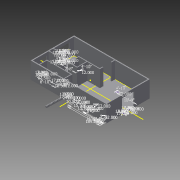
# Autodesk Inventor part: West_Test_Structure_2nd_Floor_Devices
Saved by Autodesk Inventor 2013 SP2 (Build 170200200, 200)
## iProperties
Created: 2013-07-10
Part Number: West_Test_Structure_2nd_Floor_Devices
Material: Generic
Document SubType Name: Modeling
Designer: jmw3
Density: 1 g/cm^3
Author: jmw3
Autodesk Inventor part; units mm, degrees
ref_plane "YZ Plane" through (0, 0, 0) normal (1, 0, 0) x (0, 1, 0)
ref_plane "XZ Plane" through (0, 0, 0) normal (0, 1, 0) x (-1, 0, 0)
ref_plane "XY Plane" through (0, 0, 0) normal (0, 0, 1) x (1, 0, 0)
sketch "Sketch1" plane through (0, 0, 0) normal (0, 0, 1) x (1, 0, 0)
  line L0 (-5588, 3200.4) -> (5588, 3200.4)
  line L1 (5588, -3200.4) -> (-5588, -3200.4)
  line L2 (-3958.3754, 3048) -> (-719.8754, 3048)
  line L3 (5435.6, 914.4) -> (5588, 914.4)
  line L4 (5588, -914.4) -> (5435.6, -914.4)
  line L5 (-4072.6754, 3048) -> (-605.5754, 3048)
  line L6 (5588, 3200.4) -> (5588, 914.4)
  line L7 (5588, -914.4) -> (5588, -3200.4)
  line L8 (5435.6, 3048) -> (5435.6, 914.4)
  line L9 (5435.6, -914.4) -> (5435.6, -3048)
  line L10 (-5588, 894.5564) -> (-5588, 3200.4)
  line L11 (-5435.6, 76.2) -> (-5435.6, 3048)
  line L12 (0, -4480.56) -> (0, 4480.56) projected
  line L13 (-7823.2, 0) -> (7823.2, 0) projected
  line L14 (-863.6, -3048) -> (-863.6, -2006.6)
  line L15 (-863.6, -2006.6) -> (-4381.5, -2006.6)
  line L16 (-4495.8, -2006.6) -> (-4495.8, -3048)
  line L17 (-5435.6, 76.2) -> (-3581.4, 76.2)
  line L18 (-3581.4, 76.2) -> (-3581.4, -685.8)
  line L19 (-3581.4, -685.8) -> (-5435.6, -685.8)
  line L20 (-5435.6, -571.5) -> (-5435.6, -38.1)
  line L21 (-5435.6, -38.1) -> (-3695.7, -38.1)
  line L22 (-3695.7, -38.1) -> (-3695.7, -571.5)
  line L23 (-3695.7, -571.5) -> (-5435.6, -571.5)
  line L24 (-5435.6, -571.5) -> (-5435.6, -38.1)
  line L25 (-5588, -965.2) -> (-5435.6, -965.2)
  line L26 (-5435.6, -1879.6) -> (-5588, -1879.6)
  line L27 (-5435.6, -3048) -> (-5435.6, -1879.6)
  line L28 (-5588, -3200.4) -> (-5588, -1879.6)
  line L29 (-5588, -965.2) -> (-5588, 914.4)
  line L30 (-2590.8, 914.4) -> (-1377.4097, 914.4)
  line L31 (-1244.6, 800.1) -> (-1244.6, -685.8)
  line L32 (-1244.6, -685.8) -> (-2590.8, -685.8)
  line L33 (-2590.8, -685.8) -> (-2590.8, 914.4)
  line L34 (-1377.4097, 914.4) -> (508, 914.4)
  line L35 (622.3, 952.5) -> (622.3, 800.1)
  line L36 (622.3, 800.1) -> (-1244.6, 800.1)
  line L37 (508, 914.4) -> (508, 1314.45)
  line L38 (508, 1314.45) -> (622.3, 1314.45)
  line L39 (622.3, 1314.45) -> (622.3, 800.1)
  line L40 (622.3, 3048) -> (622.3, 2533.65)
  line L41 (622.3, 2533.65) -> (508, 2533.65)
  line L42 (508, 2533.65) -> (508, 3048)
  line L43 (-2476.5, 800.1) -> (-1358.9, 800.1)
  line L44 (-1358.9, 800.1) -> (-1358.9, -571.5)
  line L45 (-1358.9, -571.5) -> (-2476.5, -571.5)
  line L46 (-2476.5, -571.5) -> (-2476.5, 800.1)
  line L47 (-749.3, -3048) -> (-749.3, -1892.3)
  line L48 (-749.3, -1892.3) -> (-4495.8, -1892.3)
  line L49 (-4495.8, -1892.3) -> (-4495.8, -2006.6)
  line L50 (-5435.6, 3048) -> (508, 3048)
  line L51 (622.3, 3048) -> (5435.6, 3048)
  line L52 (-4381.5, -2006.6) -> (-4381.5, -3048)
  line L53 (-863.6, -2006.6) -> (-1060.3581, -2006.6)
  line L54 (-5435.6, -965.2) -> (-5435.6, -685.8)
  line L55 (-5435.6, -571.5) -> (-5435.6, -38.1)
  line L56 (-4495.8, -3048) -> (-5435.6, -3048)
  line L57 (5435.6, -3048) -> (-749.3, -3048)
  line L58 (-863.6, -3048) -> (-4381.5, -3048)
  line L59 (880.3246, -3048) -> (-749.3, -3048)
  line L60 (-5435.6, -38.1) -> (-5435.6, -571.5)
  line L61 (-5435.6, -685.8) -> (-5435.6, -965.2)
  line L62 (-5435.6, -685.8) -> (-3581.4, -685.8)
  line L63 (-5435.6, 76.2) -> (-3581.4, 76.2)
  line L64 (-5435.6, 76.2) -> (-5435.6, 3048)
  line L65 (-5435.6, -685.8) -> (-5435.6, -965.2)
  line L66 (-5435.6, -965.2) -> (-5588, -965.2)
  line L67 (-5588, -965.2) -> (-5588, 3200.4)
  line L68 (-5435.6, 3048) -> (-5435.6, 76.2)
  line L69 (-5435.6, 76.2) -> (-3581.4, 76.2)
  line L70 (-3581.4, 76.2) -> (-3581.4, -685.8)
  line L71 (-3581.4, -685.8) -> (-5435.6, -685.8)
  line L72 (-5435.6, -571.5) -> (-3695.7, -571.5)
  line L73 (-3695.7, -571.5) -> (-3695.7, -38.1)
  line L74 (-3695.7, -38.1) -> (-5435.6, -38.1)
  line L75 (-5435.6, -38.1) -> (-5435.6, -571.5)
  dimension "d14" = 1828.8
  dimension "d90" = 6299.2
  dimension "d94" = 114.3
  dimension "d95" = 114.3
  dimension "d96" = 114.3
  dimension "d99" = 914.4
  dimension "d100" = 152.4
  dimension "d102" = 939.8
  dimension "d104" = 990.6
  dimension "d105" = 114.3
  dimension "d106" = 114.3
  dimension "d107" = 114.3
  dimension "d108" = 114.3
  dimension "d109" = 114.3
  dimension "d110" = 6680.2
  dimension "d112" = 1219.2
  dimension "d120" = 152.4
  dimension "d122" = 2971.8
  dimension "d123" = 2286
  dimension "d124" = 5943.6
  dimension "d125" = 114.3
  dimension "d127" = 114.3
  dimension "d128" = 6400.8
  dimension "d129" = 152.4
  dimension "d130" = 1168.4
  dimension "d131" = 1041.4
  dimension "d132" = 114.3
  dimension "d133" = 1854.2
  dimension "d134" = 2362.2
  dimension "d135" = 10871.2
  dimension "d236" = 2133.6
  dimension "d237" = 514.35
  dimension "d238" = 114.3
  constraints: 148 end point, 38 parallel, 28 perpendicular, 26 collinear, 12 horizontal, 3 point on line, 3 other
  measures "d14" distance between parallel lines of L4 L3
  measures "d90" distance between parallel lines of L9 L14
  measures "d94" distance between parallel lines of L19 L23
  measures "d95" distance between parallel lines of L18 L22
  measures "d96" distance between parallel lines of L17 L21
  measures "d99" distance between parallel lines of L25 L26
  measures "d100" distance between parallel lines of L10 L11
  measures "d102" distance between parallel lines of L27 L16
  measures "d104" distance between parallel lines of L18 L33
  measures "d105" distance between parallel lines of L33 L46
  measures "d106" distance between parallel lines of L31 L44
  measures "d107" distance between parallel lines of L32 L45
  measures "d108" distance between parallel lines of L30 L43
  measures "d109" distance between parallel lines of L39 L37
  measures "d110" distance between parallel lines of L8 L31
  measures "d112" distance from line of L38.end L41
  measures "d120" distance between parallel lines of L50 L0
  measures "d122" distance between parallel lines of L50 L17
  measures "d123" distance between parallel lines of L1 L4
  measures "d124" distance between parallel lines of L11 L37
  measures "d125" distance between parallel lines of L16 L52
  measures "d127" distance between parallel lines of L14 L47
  measures "d128" distance between parallel lines of L1 L0
  measures "d129" distance between parallel lines of L1 L57
  measures "d130" distance between parallel lines of L56 L26
  measures "d131" distance between parallel lines of L58 L15
  measures "d132" distance between parallel lines of L15 L48
  measures "d133" distance between parallel lines of L54 L18
  measures "d134" distance between parallel lines of L56 L19
  measures "d135" distance between parallel lines of L9 L27
  measures "d236" distance between parallel lines of L50 L30
  measures "d237" distance between parallel lines of L36 L38
  measures "d238" distance of L40.end L41.end
extrude "Extrusion7" add sketch "Sketch1" along normal blind 2463.8 contours L57 L9 L4 L7 L1 L12 | L12 L1 L28 L26 L27 L56 L16 L49 L48 L47 L57 | L0 L12 L50 L5 L2 L11 L17 L18 L13 L29 L10 | L0 L6 L3 L8 L51 L40 L41 L42 L50 L12 | L34 L37 L38 L39 L35 L36 L12 | L12 L36 L31 L13 L44 L43 L46 L33 L30 L34 | L13 L18 L19 L54 L25 L29 | L13 L46 L45 L44 L31 L32 L33
sketch "Sketch4" plane through (0, 0, 0) normal (0, 0, -1) x (-1, 0, 0)
  line L0 (4381.5, -3048) -> (863.6, -3048) projected
  line L1 (863.6, -3048) -> (863.6, -2006.6) projected
  line L2 (863.6, -2006.6) -> (4381.5, -2006.6) projected
  line L3 (4381.5, -2006.6) -> (4381.5, -3048) projected
  line L4 (-5435.6, -3048) -> (749.3, -3048) projected
  line L5 (-5435.6, -914.4) -> (-5435.6, -3048) projected
  line L6 (-5588, -914.4) -> (-5435.6, -914.4) projected
  line L7 (-5588, -3200.4) -> (-5588, -914.4) projected
  line L8 (5588, -3200.4) -> (-5588, -3200.4) projected
  line L9 (5588, -1879.6) -> (5588, -3200.4) projected
  line L10 (5435.6, -1879.6) -> (5588, -1879.6) projected
  line L11 (5435.6, -3048) -> (5435.6, -1879.6) projected
  line L12 (4495.8, -3048) -> (5435.6, -3048) projected
  line L13 (4495.8, -1892.3) -> (4495.8, -3048) projected
  line L14 (749.3, -1892.3) -> (4495.8, -1892.3) projected
  line L15 (749.3, -3048) -> (749.3, -1892.3) projected
  line L16 (3695.7, -571.5) -> (3695.7, -38.1) projected
  line L17 (3695.7, -38.1) -> (5435.6, -38.1) projected
  line L18 (5435.6, -38.1) -> (5435.6, -571.5) projected
  line L19 (5435.6, -571.5) -> (3695.7, -571.5) projected
  line L20 (5435.6, 3048) -> (-508, 3048) projected
  line L21 (5435.6, 76.2) -> (5435.6, 3048) projected
  line L22 (3581.4, 76.2) -> (5435.6, 76.2) projected
  line L23 (3581.4, -685.8) -> (3581.4, 76.2) projected
  line L24 (5435.6, -685.8) -> (3581.4, -685.8) projected
  line L25 (5435.6, -965.2) -> (5435.6, -685.8) projected
  line L26 (5588, -965.2) -> (5435.6, -965.2) projected
  line L27 (5588, 3200.4) -> (5588, -965.2) projected
  line L28 (-5588, 3200.4) -> (5588, 3200.4) projected
  line L29 (-5588, 914.4) -> (-5588, 3200.4) projected
  line L30 (-5435.6, 914.4) -> (-5588, 914.4) projected
  line L31 (-5435.6, 3048) -> (-5435.6, 914.4) projected
  line L32 (-622.3, 3048) -> (-5435.6, 3048) projected
  line L33 (-622.3, 2533.65) -> (-622.3, 3048) projected
  line L34 (-508, 2533.65) -> (-622.3, 2533.65) projected
  line L35 (-508, 3048) -> (-508, 2533.65) projected
  line L36 (1358.9, -571.5) -> (1358.9, 800.1) projected
  line L37 (1358.9, 800.1) -> (2476.5, 800.1) projected
  line L38 (2476.5, 800.1) -> (2476.5, -571.5) projected
  line L39 (2476.5, -571.5) -> (1358.9, -571.5) projected
  line L40 (2590.8, 914.4) -> (-508, 914.4) projected
  line L41 (-508, 914.4) -> (-508, 1314.45) projected
  line L42 (-508, 1314.45) -> (-622.3, 1314.45) projected
  line L43 (-622.3, 1314.45) -> (-622.3, 800.1) projected
  line L44 (-622.3, 800.1) -> (1244.6, 800.1) projected
  line L45 (1244.6, 800.1) -> (1244.6, -685.8) projected
  line L46 (1244.6, -685.8) -> (2590.8, -685.8) projected
  line L47 (2590.8, -685.8) -> (2590.8, 914.4) projected
  line L48 (-5588, 3200.4) -> (5588, 3200.4)
  line L49 (5588, 3200.4) -> (5588, -2006.6)
  line L50 (5588, -2006.6) -> (-5588, -2006.6)
  line L51 (-5588, -2006.6) -> (-5588, 3200.4)
  line L52 (-5588, -2006.6) -> (863.6, -2006.6)
  line L53 (863.6, -2006.6) -> (863.6, -3200.4)
  line L54 (863.6, -3200.4) -> (-5588, -3200.4)
  line L55 (-5588, -3200.4) -> (-5588, -2006.6)
  line L56 (4381.5, -2006.6) -> (5588, -2006.6)
  line L57 (5588, -2006.6) -> (5588, -3200.4)
  line L58 (5588, -3200.4) -> (4381.5, -3200.4)
  line L59 (4381.5, -3200.4) -> (4381.5, -2006.6)
  line L60 (4381.5, -3048) -> (863.6, -3048)
  line L61 (863.6, -3048) -> (863.6, -3200.4)
  line L62 (863.6, -3200.4) -> (4381.5, -3200.4)
  line L63 (4381.5, -3200.4) -> (4381.5, -3048)
  line L64 (863.6, -3200.4) -> (4381.5, -3200.4)
  line L65 (4381.5, -3200.4) -> (4381.5, -2895.6)
  line L66 (4381.5, -2895.6) -> (863.6, -2895.6)
  line L67 (863.6, -2895.6) -> (863.6, -3200.4)
  point P0 (0, 0)
  dimension "d192" = 889
  constraints: 40 end point, 10 parallel, 5 horizontal, 5 perpendicular, 3 point on line
  measures "d192" distance between parallel lines of L66 L2
extrude "Extrusion8" add sketch "Sketch4" against normal blind 25.4 contours L59 L8 L53 L0 | L3 L50 L13 L12 L11 L9 L8 L59 | L53 L8 L7 L50 L5 L4 L15 L1 | L2 L50 L15 L14 L13 | L50 L11 L12 L13 | L13 L14 L15 L50 L5 L6 L51 L30 L31 L32 L33 L34 L35 L20 L21 L22 L23 L24 L25 L26 L49 L10 L11 | L50 L11 L10 L9 | L15 L4 L5 L50 | L7 L6 L5 L50 | L26 L25 L24 L23 L22 L21 L20 L35 L34 L33 L32 L31 L30 L29 L28 L27 | L16 L17 L18 L19 | L36 L37 L38 L39 | L47 L46 L45 L44 L43 L42 L41 L40
sketch "Sketch5" plane through (-749.3, -3048, 2463.8) normal (1, 0, 0) x (0, 0, -1)
  line L0 (2438.4, 0) -> (2438.4, 1155.7) projected
  line L1 (2438.4, 1155.7) -> (0, 1155.7) projected
  line L2 (2438.4, 114.3) -> (406.4, 114.3)
  line L3 (406.4, 114.3) -> (406.4, 927.1)
  line L4 (406.4, 927.1) -> (2438.4, 927.1)
  line L5 (2438.4, 927.1) -> (2438.4, 114.3)
  line L6 (2438.4, 165.1) -> (457.2, 165.1)
  line L7 (457.2, 165.1) -> (457.2, 876.3)
  line L8 (457.2, 876.3) -> (2438.4, 876.3)
  line L9 (2438.4, 876.3) -> (2438.4, 165.1)
  point P0 (2463.8, 3048)
  dimension "d140" = 2032
  dimension "d142" = 228.6
  dimension "d143" = 812.8
  dimension "d144" = 1981.2
  dimension "d145" = 711.2
  dimension "d146" = 50.8
  constraints: 16 end point, 4 parallel, 2 horizontal, 2 perpendicular, 2 point on line
  measures "d140" distance between parallel lines of L5 L3
  measures "d142" distance between parallel lines of L1 L4
  measures "d143" distance between parallel lines of L4 L2
  measures "d144" distance between parallel lines of L9 L7
  measures "d145" distance between parallel lines of L6 L8
  measures "d146" distance between parallel lines of L2 L6
extrude "Extrusion9" cut sketch "Sketch5" against normal blind 50.8 contours L2 L3 L4 L0 L8 L7 L6
extrude "Extrusion10" cut sketch "Sketch5" against normal up to surface (114.3 mm away) contours L6 L7 L8 L0
sketch "Sketch6" plane through (0, 0, 2463.8) normal (0, 0, 1) x (1, 0, 0)
  line L0 (-3695.7, -38.1) -> (-3695.7, -571.5) projected
  line L1 (-3695.7, -571.5) -> (-5435.6, -571.5) projected
  line L2 (-5435.6, -571.5) -> (-5435.6, -38.1) projected
  line L3 (-5435.6, -38.1) -> (-3695.7, -38.1) projected
  line L4 (-5435.6, 3048) -> (508, 3048) projected
  line L5 (508, 3048) -> (508, 2533.65) projected
  line L6 (508, 2533.65) -> (622.3, 2533.65) projected
  line L7 (622.3, 2533.65) -> (622.3, 3048) projected
  line L8 (622.3, 3048) -> (5435.6, 3048) projected
  line L9 (5435.6, 3048) -> (5435.6, 914.4) projected
  line L10 (5435.6, 914.4) -> (5588, 914.4) projected
  line L11 (5588, 914.4) -> (5588, 3200.4) projected
  line L12 (5588, 3200.4) -> (-5588, 3200.4) projected
  line L13 (-5588, 3200.4) -> (-5588, -965.2) projected
  line L14 (-5588, -965.2) -> (-5435.6, -965.2) projected
  line L15 (-5435.6, -965.2) -> (-5435.6, -685.8) projected
  line L16 (-5435.6, -685.8) -> (-3581.4, -685.8) projected
  line L17 (-3581.4, -685.8) -> (-3581.4, 76.2) projected
  line L18 (-3581.4, 76.2) -> (-5435.6, 76.2) projected
  line L19 (-5435.6, 76.2) -> (-5435.6, 3048) projected
  line L20 (-1358.9, 800.1) -> (-1358.9, -571.5) projected
  line L21 (-1358.9, -571.5) -> (-2476.5, -571.5) projected
  line L22 (-2476.5, -571.5) -> (-2476.5, 800.1) projected
  line L23 (-2476.5, 800.1) -> (-1358.9, 800.1) projected
  line L24 (508, 914.4) -> (-2590.8, 914.4) projected
  line L25 (-2590.8, 914.4) -> (-2590.8, -685.8) projected
  line L26 (-2590.8, -685.8) -> (-1244.6, -685.8) projected
  line L27 (-1244.6, -685.8) -> (-1244.6, 800.1) projected
  line L28 (-1244.6, 800.1) -> (622.3, 800.1) projected
  line L29 (622.3, 800.1) -> (622.3, 1314.45) projected
  line L30 (622.3, 1314.45) -> (508, 1314.45) projected
  line L31 (508, 1314.45) -> (508, 914.4) projected
  line L32 (5435.6, 914.4) -> (5588, 914.4)
  line L33 (5588, 914.4) -> (5588, -914.4)
  line L34 (5588, -914.4) -> (5435.6, -914.4)
  line L35 (5435.6, -914.4) -> (5435.6, 914.4)
  line L36 (-5588, -965.2) -> (-5435.6, -965.2)
  line L37 (-5435.6, -965.2) -> (-5435.6, -1879.6)
  line L38 (-5435.6, -1879.6) -> (-5588, -1879.6)
  line L39 (-5588, -1879.6) -> (-5588, -965.2)
  point P0 (0, 0)
  constraints: 16 end point, 4 parallel, 2 horizontal, 2 perpendicular
extrude "Extrusion11" add sketch "Sketch6" against normal blind 406.4 contours L37 L38 L39 L14 | L10 L33 L34 L35
sketch "Sketch7" plane through (-5435.6, 76.2, 2463.8) normal (1, 0, 0) x (0, 0, -1)
  line L0 (2438.4, 0) -> (2438.4, 2971.8) projected
  line L1 (2438.4, 2971.8) -> (0, 2971.8) projected
  line L2 (431.8, 647.7) -> (1346.2, 647.7)
  line L3 (1346.2, 647.7) -> (1346.2, 2324.1)
  line L4 (1346.2, 2324.1) -> (431.8, 2324.1)
  line L5 (431.8, 2324.1) -> (431.8, 647.7)
  point P0 (2463.8, -76.2)
  dimension "d153" = 1676.4
  dimension "d155" = 914.4
  dimension "d156" = 1092.2
  dimension "d157" = 647.7
  constraints: 8 end point, 2 parallel, 1 horizontal, 1 perpendicular
  measures "d153" distance between parallel lines of L2 L4
  measures "d155" distance between parallel lines of L5 L3
  measures "d156" distance between parallel lines of L0 L3
  measures "d157" distance between parallel lines of L1 L4
extrude "Extrusion12" cut sketch "Sketch7" against normal up to surface (152.4 mm away)
sketch "Sketch9" plane through (-863.6, -3048, 2463.8) normal (-1, 0, 0) x (0, 0, 1)
  line L0 (-2463.8, 0) -> (-2438.4, 0)
  line L1 (-2438.4, 0) -> (-2438.4, 152.4)
  line L2 (-2438.4, 152.4) -> (-2463.8, 152.4)
  line L3 (-2463.8, 152.4) -> (-2463.8, 0)
  point P0 (-2463.8, 3048)
  dimension "d193" = 152.4
  constraints: 8 end point, 2 parallel, 1 horizontal, 1 perpendicular
  measures "d193" distance between parallel lines of L2 L0
extrude "Extrusion14" add sketch "Sketch9" along normal up to surface (3517.9 mm away)
sketch "Sketch11" plane through (0, 0, 2057.4) normal (0, 0, -1) x (-1, 0, 0)
  line L0 (-5435.6, -914.4) -> (-5435.6, 914.4) projected
  line L1 (-5588, 914.4) -> (-5588, -914.4) projected
  line L2 (7823.2, 0) -> (-7823.2, 0) projected
  line L3 (-5588, 12.7) -> (-5435.6, 12.7)
  line L4 (-5435.6, 12.7) -> (-5435.6, -12.7)
  line L5 (-5435.6, -12.7) -> (-5588, -12.7)
  line L6 (-5588, -12.7) -> (-5588, 12.7)
  point P0 (0, 0)
  dimension "d230" = 25.4
  constraints: 8 end point, 2 parallel, 2 point on line, 1 horizontal, 1 perpendicular, 1 other
  measures "d230" distance between parallel lines of L5 L3
extrude "Extrusion16" add sketch "Sketch11" along normal blind 25.4
sketch "Sketch10" plane through (-4381.5, -2006.6, 2463.8) normal (0, -1, 0) x (1, 0, 0)
  line L0 (3517.9, -2463.8) -> (3517.9, 0) projected
  line L1 (0, 0) -> (3517.9, 0) projected
  line L2 (3632.2, -2438.4) -> (-114.3, -2438.4) projected
  line L3 (-114.3, -2438.4) -> (-114.3, 0) projected
  line L4 (3632.2, 0) -> (-114.3, 0) projected
  line L5 (3632.2, -2438.4) -> (3632.2, 0) projected
  line L6 (850.9, -5016.5) -> (1041.4, -5016.5)
  line L7 (1041.4, -5016.5) -> (1041.4, -4832.35)
  line L8 (1041.4, -4832.35) -> (914.4, -4832.35)
  line L9 (1041.4, -4832.35) -> (1231.9, -4832.35)
  line L10 (1231.9, -4832.35) -> (1231.9, -4648.2)
  line L11 (1231.9, -4648.2) -> (1041.4, -4648.2)
  line L12 (1041.4, -4648.2) -> (1041.4, -4832.35)
  line L13 (1612.9, -4464.05) -> (1612.9, -4279.9)
  line L14 (1422.4, -4648.2) -> (1422.4, -4464.05)
  line L15 (1422.4, -4464.05) -> (1612.9, -4464.05)
  line L16 (1612.9, -4279.9) -> (1422.4, -4279.9)
  line L17 (1422.4, -4279.9) -> (1422.4, -4464.05)
  line L18 (1231.9, -4648.2) -> (1422.4, -4648.2)
  line L19 (1422.4, -4464.05) -> (1231.9, -4464.05)
  line L20 (1231.9, -4464.05) -> (1231.9, -4648.2)
  line L21 (2184.4, -3911.6) -> (2184.4, -3727.45)
  line L22 (2184.4, -3543.3) -> (2184.4, -3727.45)
  line L23 (2184.4, -3727.45) -> (2374.9, -3727.45)
  line L24 (2374.9, -3543.3) -> (2184.4, -3543.3)
  line L25 (1993.9, -3727.45) -> (1993.9, -3911.6)
  line L26 (1993.9, -3911.6) -> (2184.4, -3911.6)
  line L27 (2184.4, -3727.45) -> (1993.9, -3727.45)
  line L28 (2374.9, -3727.45) -> (2374.9, -3543.3)
  line L29 (1993.9, -4095.75) -> (1993.9, -3911.6)
  line L30 (1993.9, -3911.6) -> (1803.4, -3911.6)
  line L31 (1803.4, -4095.75) -> (1993.9, -4095.75)
  line L32 (1803.4, -3911.6) -> (1803.4, -4095.75)
  line L33 (1803.4, -4279.9) -> (1803.4, -4095.75)
  line L34 (1803.4, -4095.75) -> (1612.9, -4095.75)
  line L35 (1612.9, -4279.9) -> (1803.4, -4279.9)
  line L36 (1612.9, -4095.75) -> (1612.9, -4279.9)
  line L37 (2755.9, -3175) -> (2946.4, -3175)
  line L38 (2946.4, -3175) -> (2946.4, -2990.85)
  line L39 (2946.4, -2806.7) -> (2946.4, -2990.85)
  line L40 (2946.4, -2990.85) -> (3136.9, -2990.85)
  line L41 (3136.9, -2806.7) -> (2946.4, -2806.7)
  line L42 (3136.9, -2990.85) -> (3136.9, -2806.7)
  line L43 (3136.9, -2622.55) -> (3136.9, -2806.7)
  line L44 (3136.9, -2806.7) -> (3327.4, -2806.7)
  line L45 (3327.4, -2622.55) -> (3136.9, -2622.55)
  line L46 (3327.4, -2806.7) -> (3327.4, -2622.55)
  line L47 (2374.9, -3359.15) -> (2374.9, -3543.3)
  line L48 (2374.9, -3543.3) -> (2565.4, -3543.3)
  line L49 (2565.4, -3543.3) -> (2565.4, -3359.15)
  line L50 (2565.4, -3359.15) -> (2374.9, -3359.15)
  line L51 (2565.4, -3175) -> (2565.4, -3359.15)
  line L52 (2565.4, -3359.15) -> (2755.9, -3359.15)
  line L53 (2755.9, -3175) -> (2565.4, -3175)
  line L54 (2755.9, -3359.15) -> (2755.9, -3175)
  line L55 (2755.9, -2990.85) -> (2755.9, -3175)
  line L56 (2946.4, -2990.85) -> (2755.9, -2990.85)
  line L57 (3327.4, -2622.55) -> (3517.9, -2622.55)
  line L58 (3517.9, -2622.55) -> (3517.9, -2438.4)
  line L59 (3517.9, -2438.4) -> (3327.4, -2438.4)
  line L60 (3327.4, -2438.4) -> (3327.4, -2622.55)
  line L61 (3136.9, -2762.25) -> (3327.4, -2762.25)
  line L62 (1041.4, -4832.35) -> (850.9, -4832.35)
  line L63 (850.9, -4832.35) -> (850.9, -5016.5)
  line L64 (1041.4, -5016.5) -> (1041.4, -4832.35)
  line L65 (850.9, -5016.5) -> (660.4, -5016.5)
  line L66 (660.4, -5016.5) -> (660.4, -5200.65)
  line L67 (660.4, -5200.65) -> (850.9, -5200.65)
  line L68 (850.9, -5200.65) -> (850.9, -5016.5)
  point P0 (4381.5, -2463.8)
  dimension "d197" = 184.15
  dimension "d198" = 190.5
  dimension "d199" = 184.15
  dimension "d200" = 190.5
  dimension "d201" = 184.15
  dimension "d202" = 190.5
  dimension "d203" = 184.15
  dimension "d204" = 190.5
  dimension "d205" = 184.15
  dimension "d206" = 190.5
  dimension "d207" = 184.15
  dimension "d208" = 190.5
  dimension "d209" = 184.15
  dimension "d210" = 190.5
  dimension "d211" = 184.15
  dimension "d212" = 190.5
  dimension "d213" = 184.15
  dimension "d214" = 190.5
  dimension "d215" = 184.15
  dimension "d216" = 190.5
  dimension "d217" = 184.15
  dimension "d218" = 190.5
  dimension "d219" = 184.15
  dimension "d220" = 190.5
  dimension "d221" = 184.15
  dimension "d222" = 184.15
  dimension "d223" = 190.5
  dimension "d224" = 190.5
  dimension "d225" = 190.5
  dimension "d226" = 184.15
  constraints: 127 end point, 31 parallel, 16 horizontal, 16 perpendicular, 14 collinear, 2 point on line
  measures "d197" distance between parallel lines of L8 L6
  measures "d198" distance between parallel lines of L10 L12
  measures "d199" distance between parallel lines of L11 L9
  measures "d200" distance between parallel lines of L20 L14
  measures "d201" distance between parallel lines of L19 L18
  measures "d202" distance between parallel lines of L13 L17
  measures "d203" distance between parallel lines of L16 L15
  measures "d204" distance between parallel lines of L36 L33
  measures "d205" distance between parallel lines of L34 L35
  measures "d206" distance between parallel lines of L29 L32
  measures "d207" distance between parallel lines of L30 L31
  measures "d208" distance between parallel lines of L25 L21
  measures "d209" distance between parallel lines of L27 L26
  measures "d210" distance between parallel lines of L28 L22
  measures "d211" distance between parallel lines of L24 L23
  measures "d212" distance between parallel lines of L49 L47
  measures "d213" distance between parallel lines of L50 L48
  measures "d214" distance between parallel lines of L51 L54
  measures "d215" distance between parallel lines of L53 L52
  measures "d216" distance between parallel lines of L38 L55
  measures "d217" distance between parallel lines of L56 L37
  measures "d218" distance between parallel lines of L39 L42
  measures "d219" distance between parallel lines of L41 L40
  measures "d220" distance between parallel lines of L46 L43
  measures "d221" distance between parallel lines of L45 L44
  measures "d222" distance between parallel lines of L57 L59
  measures "d223" distance between parallel lines of L60 L58
  measures "d224" distance between parallel lines of L63 L64
  measures "d225" distance between parallel lines of L68 L66
  measures "d226" distance between parallel lines of L65 L67
extrude "Extrusion15" add sketch "Sketch10" along normal blind 889 contours L58 L57 L60 L2 L0 | L68 L67 L66 L65 | L7 L6 L63 L62 L8 | L10 L9 L12 L11 | L14 L18 L20 L19 | L13 L15 L17 L16 | L33 L35 L36 L34 | L29 L31 L32 L30 | L21 L26 L25 L27 | L28 L23 L22 L24 | L49 L48 L47 L50 | L54 L52 L51 L53 | L38 L37 L55 L56 | L42 L40 L39 L41 | L46 L61 L43 L45
sketch "Sketch12" plane through (0, 0, 25.4) normal (0, 0, 1) x (1, 0, 0)
  line L0 (-1054.1, -2895.6) -> (-863.6, -2895.6)
  line L1 (-863.6, -2895.6) -> (-863.6, -2006.6)
  line L2 (-863.6, -2006.6) -> (-1054.1, -2006.6)
  line L3 (-1054.1, -2006.6) -> (-1054.1, -2895.6)
  point P0 (0, 0)
  constraints: 8 end point, 2 parallel, 1 horizontal, 1 perpendicular
extrude "Extrusion17" cut sketch "Sketch12" against normal blind 0.0254
sketch "Sketch13" plane through (0, 0, 25.4) normal (0, 0, 1) x (1, 0, 0)
  line L0 (-863.6, -2171.7) -> (-863.6, -2882.9) projected
  line L1 (5435.6, -3048) -> (-749.3, -3048) projected
  line L2 (5435.6, -914.4) -> (5435.6, -3048) projected
  line L3 (5588, -914.4) -> (5435.6, -914.4) projected
  line L4 (5435.6, 914.4) -> (5588, 914.4) projected
  line L5 (5435.6, 3048) -> (5435.6, 914.4) projected
  line L6 (622.3, 3048) -> (5435.6, 3048) projected
  line L7 (-5435.6, 3048) -> (508, 3048) projected
  line L8 (-5435.6, 76.2) -> (-5435.6, 3048) projected
  line L9 (-3581.4, -685.8) -> (-3581.4, 76.2) projected
  line L10 (-5435.6, -965.2) -> (-5435.6, -685.8) projected
  line L11 (-5588, -965.2) -> (-5435.6, -965.2) projected
  line L12 (-5588, -965.2) -> (-5588, -1879.6) projected
  line L13 (-5435.6, -1879.6) -> (-5588, -1879.6) projected
  line L14 (-5435.6, -3048) -> (-5435.6, -1879.6) projected
  line L15 (-749.3, -1892.3) -> (-4495.8, -1892.3) projected
  line L16 (-749.3, -2120.9) -> (-749.3, -1892.3) projected
  circle A0 centre (-5435.6, -1422.4) radius 152.4
  line L17 (-5219.7, -1638.3) -> (-5651.5, -1638.3)
  circle A1 centre (-863.6, -2527.3) radius 152.4
  line L18 (-647.7, -2743.2) -> (-1079.5, -2743.2)
  line L19 (-1079.5, -2743.2) -> (-1079.5, -2311.4)
  circle A2 centre (406.4, -2527.3) radius 152.4
  circle A3 centre (4368.8, -2438.4) radius 152.4
  circle A4 centre (-3098.8, 1574.8) radius 152.4
  circle A5 centre (2387.6, -1524) radius 152.4
  circle A6 centre (2387.6, 1574.8) radius 152.4
  circle A7 centre (-5588, 1841.5) radius 152.4
  line L20 (-5372.1, 1625.6) -> (-5803.9, 1625.6)
  line L21 (-5803.9, 1625.6) -> (-5803.9, 2057.4)
  line L22 (-5803.9, 2057.4) -> (-5372.1, 1625.6)
  line L23 (-5586.4125, -963.6125) -> (-5586.4125, -965.2)
  circle A8 centre (5435.6, 457.2) radius 152.4
  line L24 (5651.5, 241.3) -> (5219.7, 241.3)
  line L25 (5219.7, 673.1) -> (5651.5, 241.3)
  line L26 (5219.7, 241.3) -> (5219.7, 673.1)
  line L27 (-7899.4, 0) -> (7835.9, 0) projected
  line L28 (0, -4480.56) -> (0, 4480.56) projected
  line L29 (-1079.5, -2311.4) -> (-647.7, -2743.2)
  line L30 (-5651.5, -1638.3) -> (-5651.5, -1206.5)
  line L31 (-5651.5, -1206.5) -> (-5219.7, -1638.3)
  line L32 (-5588, 723.9) -> (-5588, 2400.3) projected
  line L33 (-5435.6, 723.9) -> (-5588, 723.9) projected
  line L34 (-5435.6, 2400.3) -> (-5435.6, 723.9) projected
  line L35 (-5435.6, 2400.3) -> (-5588, 2400.3) projected
  circle A9 centre (-5588, 1282.7) radius 152.4
  line L36 (-5372.1, 1066.8) -> (-5803.9, 1066.8)
  line L37 (-5803.9, 1498.6) -> (-5372.1, 1066.8)
  line L38 (-5803.9, 1066.8) -> (-5803.9, 1498.6)
  circle A10 centre (-2743.2, -1422.4) radius 152.4
  line L39 (-3314.7, -1206.5) -> (-2882.9, -1206.5)
  line L40 (-2882.9, -1206.5) -> (-2882.9, -1638.3)
  line L41 (-2882.9, -1638.3) -> (-3314.7, -1638.3)
  line L42 (-3314.7, -1638.3) -> (-3314.7, -1206.5)
  line L43 (190.5, -2222.5) -> (622.3, -2222.5)
  line L44 (622.3, -2222.5) -> (622.3, -2654.3)
  line L45 (622.3, -2654.3) -> (190.5, -2654.3)
  line L46 (190.5, -2654.3) -> (190.5, -2222.5)
  circle A11 centre (2387.6, -2438.4) radius 152.4
  line L47 (2603.5, -2654.3) -> (2171.7, -2654.3)
  line L48 (2171.7, -2654.3) -> (2171.7, -2222.5)
  line L49 (2171.7, -2222.5) -> (2603.5, -2654.3)
  line L50 (5219.7, -673.1) -> (5219.7, -241.3)
  line L51 (5219.7, -241.3) -> (5651.5, -673.1)
  line L52 (5651.5, -673.1) -> (5219.7, -673.1)
  circle A12 centre (5435.6, -457.2) radius 152.4
  line L53 (2563.5764, -2133.6) -> (2739.5527, -2438.4)
  line L54 (2739.5527, -2438.4) -> (2563.5764, -2743.2)
  line L55 (2563.5764, -2743.2) -> (2211.6236, -2743.2)
  line L56 (2211.6236, -2743.2) -> (2035.6473, -2438.4)
  line L57 (2035.6473, -2438.4) -> (2211.6236, -2133.6)
  line L58 (2211.6236, -2133.6) -> (2563.5764, -2133.6)
  line L59 (-687.6236, -2222.5) -> (-511.6473, -2527.3)
  line L60 (-511.6473, -2527.3) -> (-687.6236, -2832.1)
  line L61 (-687.6236, -2832.1) -> (-1039.5764, -2832.1)
  line L62 (-1039.5764, -2832.1) -> (-1215.5527, -2527.3)
  line L63 (-1215.5527, -2527.3) -> (-1039.5764, -2222.5)
  line L64 (-1039.5764, -2222.5) -> (-687.6236, -2222.5)
  point P0 (0, 0)
  point P1 (5435.6, -457.2)
  point P2 (5435.6, 457.2)
  point P3 (-863.6, -2222.5)
  dimension "d242" = 304.8
  dimension "d246" = 457.2
  dimension "d247" = 431.8
  dimension "d248" = 431.8
  dimension "d249" = 241.3
  dimension "d251" = 304.8
  dimension "d252" = 431.8
  dimension "d253" = 431.8
  dimension "d256" = 215.9
  dimension "d257" = 304.8
  dimension "d258" = 304.8
  dimension "d259" = 304.8
  dimension "d260" = 304.8
  dimension "d261" = 304.8
  dimension "d262" = 304.8
  dimension "d263" = 431.8
  dimension "d264" = 431.8
  dimension "d265" = 215.9
  dimension "d266" = 304.8
  dimension "d267" = 431.8
  dimension "d268" = 431.8
  dimension "d269" = 215.9
  dimension "d270" = 1473.2
  dimension "d271" = 2336.8
  dimension "d272" = 1473.2
  dimension "d273" = 3048
  dimension "d274" = 1524
  dimension "d275" = 3048
  dimension "d276" = 5029.2
  dimension "d277" = 1066.8
  dimension "d278" = 609.6
  dimension "d280" = 215.9
  dimension "d281" = 558.8
  dimension "d282" = 304.8
  dimension "d283" = 431.8
  dimension "d284" = 431.8
  dimension "d285" = 215.9
  dimension "d286" = 558.8
  dimension "d287" = 304.8
  dimension "d289" = 2692.4
  dimension "d290" = 431.8
  dimension "d291" = 431.8
  dimension "d292" = 215.9
  dimension "d293" = 2120.9
  dimension "d294" = 431.8
  dimension "d295" = 431.8
  dimension "d296" = 393.7
  dimension "d297" = 4813.3
  dimension "d298" = 304.8
  dimension "d299" = 609.6
  dimension "d300" = 3048
  dimension "d301" = 431.8
  dimension "d302" = 431.8
  dimension "d303" = 393.7
  dimension "d304" = 304.8
  dimension "d305" = 431.8
  dimension "d306" = 431.8
  dimension "d307" = 215.9
  dimension "d308" = 457.2
  dimension "d309" = 457.2
  dimension "d310" = 609.6
  dimension "d311" = 609.6
  dimension "d332" = 469.9
  dimension "d333" = 520.7
  constraints: 84 end point, 19 parallel, 13 centre point, 10 midpoint, 7 point on line, 2 coincident, 2 horizontal, 2 perpendicular, 26 other
  measures "d242" diameter of A0
  measures "d246" distance from line of L13 A0.centre
  measures "d247" distance of L17.end L30.end
  measures "d248" distance of L17.start L17.end
  measures "d249" distance between parallel lines of L13 L17
  measures "d251" diameter of A1
  measures "d252" distance of L18.start L18.end
  measures "d253" distance of L18.end L19.end
  measures "d256" distance between parallel lines of L0 L19
  measures "d257" diameter of A2
  measures "d258" diameter of A3
  measures "d259" diameter of A4
  measures "d260" diameter of A5
  measures "d261" diameter of A6
  measures "d262" diameter of A7
  measures "d263" distance of L20.end L22.start
  measures "d264" distance of L20.start L20.end
  measures "d265" distance from line of A7.centre L21
  measures "d266" diameter of A8
  measures "d267" distance of L26.start L26.end
  measures "d268" distance of L25.end L26.start
  measures "d269" distance from line of A8.centre L26
  measures "d270" distance from line of L7 A4.centre
  measures "d271" distance from line of L8 A4.centre
  measures "d272" distance from line of L6 A6.centre
  measures "d273" distance from line of L5 A6.centre
  measures "d274" distance from line of L1 A5.centre
  measures "d275" distance from line of L2 A5.centre
  measures "d276" distance from line of L2 A2.centre
  measures "d277" distance from line of L2 A3.centre
  measures "d278" distance from line of L1 A3.centre
  measures "d280" distance from line of A0.centre L30
  measures "d281" distance from line of L35 A7.centre
  measures "d282" diameter of A9
  measures "d283" distance of L36.end L38.end
  measures "d284" distance of L36.start L36.end
  measures "d285" distance from line of A9.centre L38
  measures "d286" distance from line of L33 A9.centre
  measures "d287" diameter of A10
  measures "d289" distance from line of L14 A10.centre
  measures "d290" distance of L41.end L39.start
  measures "d291" distance of L39.start L39.end
  measures "d292" distance from line of A10.centre L39
  measures "d293" distance between parallel lines of L14 L42
  measures "d294" distance between parallel lines of L43 L45
  measures "d295" distance of L43.start L43.end
  measures "d296" distance between parallel lines of L1 L45
  measures "d297" distance between parallel lines of L2 L44
  measures "d298" diameter of A11
  measures "d299" distance from line of L1 A11.centre
  measures "d300" distance from line of L2 A11.centre
  measures "d301" distance of L47.end L48.end
  measures "d302" distance of L47.start L47.end
  measures "d303" distance between parallel lines of L1 L47
  measures "d304" diameter of A12
  measures "d305" distance of L50.start L50.end
  measures "d306" distance of L51.end L50.start
  measures "d307" distance from line of A12.centre L50
  measures "d308" distance from line of L3 A12.centre
  measures "d309" distance from line of L4 A8.centre
  measures "d310" distance between parallel lines of L55 L58
  measures "d311" distance between parallel lines of L61 L64
  measures "d332" distance from line of L15 A10.centre
  measures "d333" distance from line of L1 A2.centre
extrude "Extrusion18" add sketch "Sketch13" along normal blind 76.2 contours A1 L29 L0 | L0 L29 A1 | L29 A1 L0 | L0 A1 L29 | A7 L22 L32 | L32 L22 A7 | A7 L32 L22 | L22 L32 A7 | A9 L37 L32 | L32 L37 A9 | A9 L32 L37 | L32 A9 L37 | A0 L31 | A0 L31 | A2 L45 | L45 A2 | A3 | A4 | A5 | A6 | A8 L25 | L25 A8 | A10 L40 | L40 A10 | A11 L49 | L49 A11 | A12 L51 | L51 A12
extrude "Extrusion19" add sketch "Sketch13" along normal blind 50.8 contours L29 A1 L0 | L0 A1 L29 | A1 L0 L18 L19 L29 | A1 L29 L18 L0 | L22 L20 L8 | L8 L20 L32 A7 L22 | A7 L32 L22 | L22 L32 A7 | A7 L32 L20 L21 L22 | L37 L36 L8 | L8 L36 L32 A9 L37 | A9 L32 L37 | L32 A9 L37 | A9 L32 L36 L38 L37 | L31 A0 L12 | L12 L17 L30 L31 | A0 L31 L17 L12 | A0 L31 | A2 L45 | A2 L45 L46 L43 L44 | L25 A8 | A8 L25 L24 L26 | L40 A10 | A10 L40 L41 L42 L39 | L49 A11 | A11 L49 L47 L48 | L50 L51 A12 L52 | L51 A12 picked at (-796.0057, -2602.9381) picked at (-952.3828, -2576.3685) picked at (-5529.2995, 1758.7694) picked at (-5626.8195, 1747.7815) picked at (-5529.2995, 1199.9694) picked at (-5626.8195, 1188.9815) picked at (-5481.3692, -1400.3587) picked at (366.3236, -2477.213) picked at (5377.7074, 448.3062) picked at (-2884.7373, -1406.9827) picked at (2347.883, -2478.5688) picked at (5377.7074, -466.0938)
extrude "Extrusion20" add sketch "Sketch13" along normal blind 25.4 contours L64 L59 L60 L61 L0 L18 L29 A1 | L0 A1 L29 L19 L18 L61 L62 L63 L64 | L53 L54 L55 L56 L57 L58
sketch "Sketch15" plane through (-5435.6, 723.9, 1117.6) normal (0, 0, 1) x (1, 0, 0)
  line L0 (-152.4, 0) -> (-152.4, 1676.4) projected
  line L1 (0, 0) -> (-152.4, 0) projected
  line L2 (0, 1676.4) -> (-152.4, 1676.4) projected
  circle A0 centre (-152.4, 1117.6) radius 152.4
  line L3 (63.5, 901.7) -> (-368.3, 901.7)
  line L4 (-368.3, 1333.5) -> (63.5, 901.7)
  line L5 (-368.3, 901.7) -> (-368.3, 1333.5)
  line L6 (63.5, 342.9) -> (-368.3, 342.9)
  circle A1 centre (-152.4, 558.8) radius 152.4
  line L7 (-368.3, 342.9) -> (-368.3, 774.7)
  line L8 (-368.3, 774.7) -> (63.5, 342.9)
  point P0 (5435.6, -723.9)
  dimension "d318" = 304.8
  dimension "d319" = 431.8
  dimension "d320" = 431.8
  dimension "d321" = 215.9
  dimension "d322" = 304.8
  dimension "d323" = 431.8
  dimension "d324" = 431.8
  dimension "d325" = 215.9
  dimension "d326" = 558.8
  dimension "d327" = 558.8
  constraints: 12 end point, 4 parallel, 3 midpoint, 2 centre point, 1 collinear, 1 point on line
  measures "d318" diameter of A0
  measures "d319" distance of L3.end L4.start
  measures "d320" distance of L3.start L3.end
  measures "d321" distance from line of A0.centre L5
  measures "d322" diameter of A1
  measures "d323" distance of L6.end L8.start
  measures "d324" distance of L6.start L6.end
  measures "d325" distance from line of A1.centre L7
  measures "d326" distance from line of L2 A0.centre
  measures "d327" distance from line of L1 A1.centre
extrude "Extrusion21" add sketch "Sketch15" along normal blind 50.8 contours L6 L7 L8 A1 L0 | L0 A1 L8 L6 | L3 L5 L4 A0 L0 | L0 A0 L4 L3 | A1 L8 L0 | L0 L8 A1 | A0 L4 L0 | L0 L4 A0 picked at (-246.1185, 519.9805) picked at (-84.8057, 483.1619) picked at (-158.0878, 1016.3194) picked at (-84.8057, 1041.9619)
extrude "Extrusion22" add sketch "Sketch15" along normal blind 76.2 contours A1 L8 L0 | L0 L8 A1 | L8 A1 L0 | L0 A1 L8 | A0 L4 L0 | L0 L4 A0 | L4 A0 L0 | L0 A0 L4
body "Solid2"
